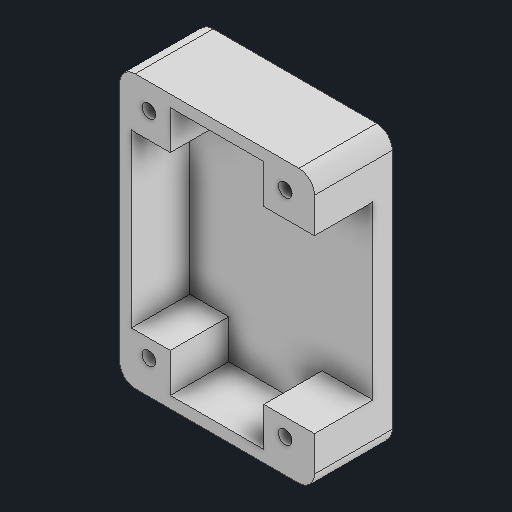
# Autodesk Inventor part: HOLDER
Saved by Autodesk Inventor 2026.2 (Build 302298010, 298A)
## iProperties
Created: 2026-04-09
Part Number: HOLDER
Material: Generic
Document SubType Name: Modeling
Designer: Cat
Density: 1 g/cm^3
Appearance: Default
Author: Cat
Autodesk Inventor part; units mm, degrees
ref_plane "YZ Plane" through (0, 0, 0) normal (1, 0, 0) x (0, 1, 0)
ref_plane "XZ Plane" through (0, 0, 0) normal (0, 1, 0) x (-1, 0, 0)
ref_plane "XY Plane" through (0, 0, 0) normal (0, 0, 1) x (1, 0, 0)
sketch "Sketch1" plane through (0, 0, 0) normal (0, 0, 1) x (1, 0, 0)
  line L0 (0, 0) -> (50, 0)
  line L1 (50, 0) -> (50, 70)
  line L2 (50, 70) -> (0, 70)
  line L3 (0, 70) -> (0, 0)
  dimension "d0" = 50
  dimension "d1" = 70
  constraints: 8 end point, 2 parallel, 1 horizontal, 1 perpendicular
  measures "d0" distance of L2.end L1.end
  measures "d1" distance of L1.end L0.end
extrude "Extrusion1" add sketch "Sketch1" along normal blind 20
sketch "Sketch2" plane through (0, 0, 20) normal (0, 0, 1) x (1, 0, 0)
  line L0 (50, 70) -> (0, 70) projected
  line L1 (0, 0) -> (50, 0) projected
  line L2 (3, 67) -> (47, 67)
  line L3 (47, 67) -> (47, 3)
  line L4 (47, 3) -> (3, 3)
  line L5 (3, 3) -> (3, 67)
  line L6 (0, 70) -> (0, 0) projected
  dimension "d4" = 44
  dimension "d5" = 64
  dimension "d6" = 3
  dimension "d7" = 3
  constraints: 8 end point, 2 parallel, 1 horizontal, 1 perpendicular
  measures "d4" distance of L2.start L2.end
  measures "d5" distance of L2.end L3.end
  measures "d6" distance between parallel lines of L2 L0
  measures "d7" distance between parallel lines of L6 L5
extrude "Extrusion2" cut sketch "Sketch2" against normal blind 15
sketch "Sketch3" plane through (0, 0, 20) normal (0, 0, 1) x (1, 0, 0)
  line L0 (50, 70) -> (0, 70) projected
  line L1 (0, 70) -> (13, 70)
  line L2 (13, 70) -> (13, 57)
  line L3 (13, 57) -> (0, 57)
  line L4 (0, 57) -> (0, 70)
  line L5 (0, 0) -> (50, 0) projected
  line L6 (0, 0) -> (13, 0)
  line L7 (13, 0) -> (13, 13)
  line L8 (13, 13) -> (0, 13)
  line L9 (0, 13) -> (0, 0)
  line L10 (50, 70) -> (37, 70)
  line L11 (37, 70) -> (37, 57)
  line L12 (37, 57) -> (50, 57)
  line L13 (50, 57) -> (50, 70)
  line L14 (50, 0) -> (37, 0)
  line L15 (37, 0) -> (37, 13)
  line L16 (37, 13) -> (50, 13)
  line L17 (50, 13) -> (50, 0)
  point P0 (37, 0)
  dimension "d10" = 13
  dimension "d11" = 13
  constraints: 32 end point, 9 parallel, 6 equal length, 4 horizontal, 4 perpendicular
  measures "d10" distance of L2.end L3.end
  measures "d11" distance of L1.end L2.end
extrude "Extrusion3" add sketch "Sketch3" against normal up to surface (15 mm away)
sketch "Sketch4" plane through (0, 0, 20) normal (0, 0, 1) x (1, 0, 0)
  line L0 (7.5, 63.5) -> (42.5, 63.5)
  line L1 (42.5, 63.5) -> (42.5, 8.5)
  line L2 (42.5, 8.5) -> (7.5, 8.5)
  line L3 (7.5, 8.5) -> (7.5, 63.5)
  circle A0 centre (7.5, 63.5) radius 1.75
  circle A1 centre (42.5, 63.5) radius 1.75
  circle A2 centre (42.5, 8.5) radius 1.75
  circle A3 centre (7.5, 8.5) radius 1.75
  line L4 (50, 70) -> (0, 70) projected
  line L5 (47, 57) -> (37, 57) projected
  line L6 (50, 0) -> (50, 70) projected
  point P0 (0, 0)
  dimension "d18" = 3.5
  dimension "d22" = 35
  dimension "d23" = 55
  dimension "d24" = 7.5
  dimension "d25" = 6.5
  constraints: 8 end point, 4 centre point, 4 coincident, 3 equal radius, 2 parallel, 1 horizontal, 1 perpendicular
  measures "d18" diameter of A1
  measures "d22" distance of L0.start A1.centre
  measures "d23" distance of L1.end A1.centre
  measures "d24" distance from line of L6 A1.centre
  measures "d25" distance between parallel lines of L4 L0
extrude "Extrusion4" cut sketch "Sketch4" against normal blind 5 contours L3 A0 L0 | L0 A0 L3 | A1 L1 L0 | L0 L1 A1 | A3 L2 L3 | L3 L2 A3 | A2 L1 L2 | L2 L1 A2
sketch "Sketch5" plane through (50, 0, 0) normal (1, 0, 0) x (0, 0, -1)
  line L0 (-20, 13) -> (-5, 13) projected
  line L1 (-20, 57) -> (-5, 57) projected
  line L2 (-5, 13) -> (-5, 57) projected
  line L3 (-20, 13) -> (-5, 13)
  line L4 (-5, 13) -> (-5, 57)
  line L5 (-5, 57) -> (-20, 57)
  line L6 (-20, 57) -> (-20, 13)
  point P0 (0, 0)
  constraints: 8 end point, 2 parallel, 1 horizontal, 1 perpendicular
extrude "Extrusion5" cut sketch "Sketch5" against normal up to surface (47 mm away)
fillet "Fillet2" radius 4 4 edges at (0, 70, 10) (50, 70, 10) (50, 0, 10) (0, 0, 10)
body "Solid1"
